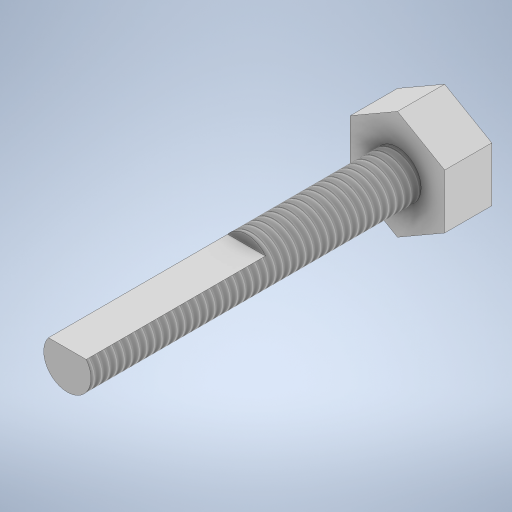
# Autodesk Inventor part: m5-screw-cut
Saved by Autodesk Inventor 2023 (Build 270158000, 158)
## iProperties
Created: 2023-06-05
Part Number: m5-screw-cut
Material: Generic
Document SubType Name: Modeling
Designer: Ronan
Density: 1 g/cm^3
Appearance: Default
Author: Ronan
Autodesk Inventor part; units mm, degrees
ref_plane "YZ Plane" through (0, 0, 0) normal (1, 0, 0) x (0, 1, 0)
ref_plane "XZ Plane" through (0, 0, 0) normal (0, 1, 0) x (-1, 0, 0)
ref_plane "XY Plane" through (0, 0, 0) normal (0, 0, 1) x (1, 0, 0)
sketch "Sketch1" plane through (0, 0, 0) normal (0, 0, 1) x (1, 0, 0)
  line L0 (5, 2.8868) -> (5, -2.8868)
  line L1 (5, 2.8868) -> (0, 5.7735)
  line L2 (-5, 2.8868) -> (0, 5.7735)
  line L3 (0, -5.7735) -> (5, -2.8868)
  line L4 (-5, 2.8868) -> (-5, -2.8868)
  line L5 (-5, -2.8868) -> (0, -5.7735)
  point P0 (0, 0)
  point P1 (0, 0)
  point P2 (0, 0)
  point P3 (0, 0)
  point P4 (0, 0)
  point P5 (0, 0)
  dimension "d0" = 120
  dimension "d1" = 120
  dimension "d2" = 120
  dimension "d3" = 120
  dimension "d4" = 120
  dimension "d5" = 120
  dimension "d6" = 10
  dimension "d7" = 5
  constraints: 12 end point, 3 coincident, 2 vertical
  measures "d0" angle of L3 L0
  measures "d1" angle of L5 L3
  measures "d2" angle of L5 L4
  measures "d3" angle of L4 L2
  measures "d4" angle of L2 L1
  measures "d5" angle of L1 L0
  measures "d6" distance between parallel lines of L0 L4
  measures "d7" distance from line of L4 point (0, 0)
extrude "Extrusion1" add sketch "Sketch1" along normal blind 5
sketch "Sketch2" plane through (0, 0, 5) normal (0, 0, 1) x (1, 0, 0)
  circle A0 centre (0, 0) radius 2.5
  dimension "d10" = 5
  constraints: 1 centre point, 1 coincident
  measures "d10" diameter of A0
extrude "Extrusion2" add sketch "Sketch2" along normal blind 35
thread "Thread1" size "M5x0.8" class "6g" standard "ANSI Metric M Profile" full length
sketch "Sketch3" plane through (0, 0, 40) normal (0, 0, 1) x (1, 0, 0)
  line L0 (0, 0) -> (0, 1.5)
  line L1 (0, 1.5) -> (2, 1.5)
  line L2 (2, 1.5) -> (-2, 1.5)
  circle A0 centre (0, 0) radius 2.5 projected
  circle A1 centre (0, 0) radius 2.5
  dimension "d15" = 1.5
  constraints: 6 end point, 1 coincident, 1 perpendicular, 1 point on line, 1 vertical, 5 other
  measures "d15" distance of L0.start L0.end
extrude "Extrusion3" cut sketch "Sketch3" against normal blind 19 contours L2 A0 L1 picked at (-1.2006, 1.6398)
body "Solid1"
